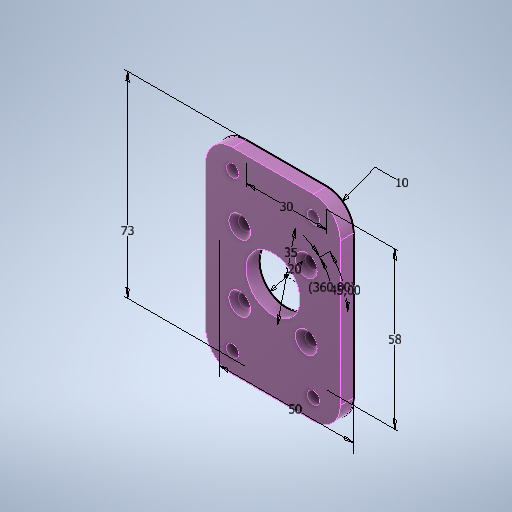
# Autodesk Inventor part: кронштейн
Saved by Autodesk Inventor 2025 (Build 290162000, 162)
## iProperties
Created: 2025-02-17
Part Number: кронштейн
Material: Сталь
Document SubType Name: Sheet Metal
Designer: volko
Density: 7.85 g/cm^3
Sheet Metal Rule: По умолчанию_мм
Appearance: Гладкий — пурпурный
Mass: 127.786 g
Surface Area: 126.326 cm^2
Volume: 16.2784 cm^3
Author: volko
Autodesk Inventor part; units mm, degrees
ref_plane "YZ Plane" through (0, 0, 0) normal (1, 0, 0) x (0, 1, 0)
ref_plane "XZ Plane" through (0, 0, 0) normal (0, 1, 0) x (-1, 0, 0)
ref_plane "XY Plane" through (0, 0, 0) normal (0, 0, 1) x (1, 0, 0)
sketch "Эскиз1" plane through (0, 0, 0) normal (0, 0, 1) x (1, 0, 0)
  line L0 (0, 0) -> (0, 36.5) construction
  line L1 (0, 36.5) -> (15, 36.5)
  line L2 (25, 26.5) -> (25, 0)
  line L3 (0, 0) -> (25, 0) construction
  arc A0 (25, 26.5) -> (15, 36.5) centre (15, 26.5) ccw
  line L4 (0, 36.5) -> (-15, 36.5)
  line L5 (-25, 26.5) -> (-25, 0)
  arc A1 (-15, 36.5) -> (-25, 26.5) centre (-15, 26.5) ccw
  circle A2 centre (0, 0) radius 10
  circle A3 centre (0, 0) radius 17.5 construction
  line L6 (0, 0) -> (12.3744, 12.3744) construction
  line L7 (-11.5586, -36.5) -> (15, -36.5)
  line L8 (25, -26.5) -> (25, 0)
  arc A4 (15, -36.5) -> (25, -26.5) centre (15, -26.5) ccw
  line L9 (-11.5586, -36.5) -> (-15, -36.5)
  arc A5 (-25, -26.5) -> (-15, -36.5) centre (-15, -26.5) ccw
  line L10 (-25, -26.5) -> (-25, 0)
  point P0 (-12.3744, 12.3744)
  point P1 (-12.3744, -12.3744)
  point P2 (12.3744, -12.3744)
  point P3 (15, 29)
  point P4 (-15, 29)
  point P5 (15, -29)
  point P6 (-15, -29)
  dimension "d6" = 35
  dimension "d4" = 50
  dimension "d5" = 20
  dimension "d8" = 45
  dimension "d42" = 73
  dimension "d43" = 10
  dimension "d46" = 360
  dimension "d50" = 30
  dimension "d53" = 58
  constraints: 22 end point, 8 point on circle, 6 symmetric about line, 6 tangent, 5 centre point, 4 coincident, 4 vertical, 3 perpendicular, 2 equal radius, 2 point on line, 1 horizontal, 1 parallel, 13 other
  measures "d4" distance between parallel lines of L2 L5
  measures "d5" diameter of A2
  measures "d8" angle of L3 L6
  measures "d42" distance between parallel lines of L9 L4
  measures "d43" radius of A0
  measures "d50" distance of point (15, 29) point (-15, 29)
  measures "d53" distance of point (15, 29) point (15, -29)
sketch "Эскиз5" plane through (-25, 3, -67) normal (0, 1, 0) x (1, 0, 0)
  line L0 (0, -64) -> (50, -64) projected
  line L1 (25, -64) -> (25, 0) construction
  line L2 (7, -58.1) -> (7, -45.9) construction
  arc A0 (9.1, -48) -> (7, -45.9) centre (7, -48) ccw
  line L3 (9.1, -48) -> (9.1, -52)
  line L4 (9.1, -52) -> (4.9, -52) construction
  arc A1 (7, -58.1) -> (9.1, -56) centre (7, -56) ccw
  line L5 (9.1, -56) -> (9.1, -52)
  arc A2 (7, -45.9) -> (4.9, -48) centre (7, -48) ccw
  line L6 (4.9, -48) -> (4.9, -52)
  line L7 (4.9, -56) -> (4.9, -52)
  arc A3 (4.9, -56) -> (7, -58.1) centre (7, -56) ccw
  line L8 (7, -21.1) -> (7, -8.9) construction
  arc A4 (9.1, -11) -> (7, -8.9) centre (7, -11) ccw
  line L9 (9.1, -11) -> (9.1, -15)
  line L10 (9.1, -15) -> (4.9, -15) construction
  line L11 (9.1, -19) -> (9.1, -15)
  arc A5 (7, -21.1) -> (9.1, -19) centre (7, -19) ccw
  arc A6 (4.9, -19) -> (7, -21.1) centre (7, -19) ccw
  line L12 (4.9, -19) -> (4.9, -15)
  line L13 (4.9, -11) -> (4.9, -15)
  arc A7 (7, -8.9) -> (4.9, -11) centre (7, -11) ccw
  line L14 (43, -58.1) -> (43, -45.9) construction
  arc A8 (45.1, -48) -> (43, -45.9) centre (43, -48) ccw
  line L15 (45.1, -48) -> (45.1, -52)
  line L16 (45.1, -52) -> (40.9, -52) construction
  line L17 (45.1, -56) -> (45.1, -52)
  arc A9 (43, -58.1) -> (45.1, -56) centre (43, -56) ccw
  arc A10 (40.9, -56) -> (43, -58.1) centre (43, -56) ccw
  line L18 (40.9, -56) -> (40.9, -52)
  line L19 (40.9, -48) -> (40.9, -52)
  arc A11 (43, -45.9) -> (40.9, -48) centre (43, -48) ccw
  line L20 (43, -21.1) -> (43, -8.9) construction
  arc A12 (45.1, -11) -> (43, -8.9) centre (43, -11) ccw
  line L21 (45.1, -11) -> (45.1, -15)
  line L22 (45.1, -15) -> (40.9, -15) construction
  line L23 (45.1, -19) -> (45.1, -15)
  arc A13 (43, -21.1) -> (45.1, -19) centre (43, -19) ccw
  arc A14 (40.9, -19) -> (43, -21.1) centre (43, -19) ccw
  line L24 (40.9, -19) -> (40.9, -15)
  line L25 (40.9, -11) -> (40.9, -15)
  arc A15 (43, -8.9) -> (40.9, -11) centre (43, -11) ccw
  line L26 (50, 0) -> (0, 0) projected
  point P0 (25, -67)
  point P1 (4.9, -50)
  point P2 (9.1, -50)
  point P3 (9.1, -13)
  point P4 (4.9, -13)
  point P5 (45.1, -50)
  point P6 (40.9, -50)
  point P7 (45.1, -13)
  point P8 (40.9, -13)
  dimension "d29" = 8
  dimension "d30" = 4.2
  dimension "d33" = 37
  dimension "d36" = 36
  dimension "d39" = 15
  constraints: 50 end point, 32 point on circle, 16 centre point, 6 symmetric about line, 4 vertical, 3 midpoint, 1 horizontal, 1 tangent, 70 other
  measures "d29" distance of A0.centre A1.centre
  measures "d30" distance of point (4.9, -50) point (9.1, -50)
  measures "d33" distance of L2.start L8.start
  measures "d36" distance of L2.start L14.start
  measures "d39" distance between parallel lines of L26 L10
extrude "Пластина2" add sketch "Эскиз1" along normal blind 5
hole "Отверстие2" at (-15, 29, 0) at (-15, -29, 0) at (15, -29, 0) at (15, 29, 0) direction (0, 0, 1) diameter 4.5 end through all countersink diameter 8 countersink angle 90
sketch "Эскиз6" plane through (0, 0, 5) normal (0, 0, 1) x (1, 0, 0)
  circle A0 centre (0, 0) radius 17.5 construction
  point P0 (12.3744, 12.3744)
  point P1 (-12.3744, 12.3744)
  point P2 (-12.3744, -12.3744)
  point P3 (12.3744, -12.3744)
  dimension "d72" = 360
  constraints: 1 coincident, 8 other
hole "Отверстие3" at (-12.3744, 12.3744, 5) at (-12.3744, -12.3744, 5) at (12.3744, -12.3744, 5) at (12.3744, 12.3744, 5) direction (0, 0, -1) diameter 4.5 end through all countersink diameter 8 countersink angle 90
sketch "Эскиз4" plane through (-25, 3, 3) normal (0, -1, 0) x (1, 0, 0)
  line L0 (50, 0) -> (0, 0)
  line L1 (0, 0) -> (0, -70)
  line L2 (0, -70) -> (50, -70)
  line L3 (50, -70) -> (50, 0)
  constraints: 6 end point, 1 horizontal, 1 perpendicular, 1 vertical
equation "\"d18\" = Толщина"
equation "\"Радиус_гибки\" = Толщина"
equation "\"Ширина_просечки\" = Толщина"
equation "\"Глубина_просечки\" = 0.5 * Толщина"
equation "\"Радиус_перехода\" = Радиус_гибки"
equation "\"Радиус_Якоби\" = Радиус_гибки"
equation "\"Размер_зазора\" = Толщина"
equation "\"Толщина\" = 5"
